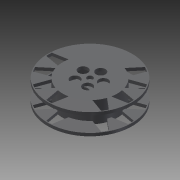
# Autodesk Inventor part: Wheel
Saved by Autodesk Inventor 2014 SP1 (Build 180222100, 222)
## iProperties
Created: 2014-11-21
Part Number: Wheel
Material: Generic
Document SubType Name: Modeling
Designer: AlecShufelt
Density: 1 g/cm^3
Appearance: Smooth - Medium Gray
Author: AlecShufelt
Autodesk Inventor part; units mm, degrees
ref_plane "YZ Plane" through (0, 0, 0) normal (1, 0, 0) x (0, 1, 0)
ref_plane "XZ Plane" through (0, 0, 0) normal (0, 1, 0) x (-1, 0, 0)
ref_plane "XY Plane" through (0, 0, 0) normal (0, 0, 1) x (1, 0, 0)
sketch "Sketch1" plane through (0, 0, 0) normal (0, 1, 0) x (-1, 0, 0)
  circle A0 centre (0, 0) radius 114.3
  dimension "d0" = 228.6
  constraints: 1 centre point, 1 coincident
  measures "d0" diameter of A0
extrude "Extrusion1" add sketch "Sketch1" along normal blind 7.9756
sketch "Sketch2" plane through (0, 7.9756, 0) normal (0, 1, 0) x (1, 0, 0)
  circle A0 centre (0, 0) radius 114.3 projected
  circle A1 centre (0, 0) radius 74.2569
  dimension "d3" = 148.5138
  constraints: 1 centre point, 1 coincident
  measures "d3" diameter of A1
extrude "Extrusion2" add sketch "Sketch2" along normal blind 41.0464 contours A1
sketch "Sketch3" plane through (0, 49.022, 0) normal (0, 1, 0) x (1, 0, 0)
  circle A0 centre (0, 0) radius 74.2569 projected
  circle A1 centre (0, 0) radius 114.3
  dimension "d6" = 228.6
  constraints: 1 centre point, 1 coincident
  measures "d6" diameter of A1
extrude "Extrusion3" add sketch "Sketch3" along normal blind 7.9756 contours A0 | A1
sketch "Sketch4" plane through (0, 56.9976, 0) normal (0, 1, 0) x (1, 0, 0)
  circle A0 centre (0, 0) radius 114.3 projected
  circle A1 centre (0, 0) radius 111.76
  circle A2 centre (0, 0) radius 74.2569
  line L0 (14.605, 72.8065) -> (7.62, 111.4999)
  line L1 (-14.605, 72.8065) -> (-7.62, 111.4999)
  line L2 (0, 0) -> (0, 82.3144)
  circle A3 centre (0, 0) radius 111.76
  circle A4 centre (0, 0) radius 74.2569
  line L3 (-23.7549, 70.3547) -> (-49.1508, 100.3718)
  line L4 (-49.0515, 55.7497) -> (-62.3491, 92.7518)
  circle A5 centre (0, 0) radius 111.76
  circle A6 centre (0, 0) radius 74.2569
  line L5 (-55.7497, 49.0515) -> (-92.7518, 62.3491)
  line L6 (-70.3547, 23.7549) -> (-100.3718, 49.1508)
  circle A7 centre (0, 0) radius 111.76
  circle A8 centre (0, 0) radius 74.2569
  line L7 (-72.8065, 14.605) -> (-111.4999, 7.62)
  line L8 (-72.8065, -14.605) -> (-111.4999, -7.62)
  circle A9 centre (0, 0) radius 111.76
  circle A10 centre (0, 0) radius 74.2569
  line L9 (-70.3547, -23.7549) -> (-100.3718, -49.1508)
  line L10 (-55.7497, -49.0515) -> (-92.7518, -62.3491)
  circle A11 centre (0, 0) radius 111.76
  circle A12 centre (0, 0) radius 74.2569
  line L11 (-49.0515, -55.7497) -> (-62.3491, -92.7518)
  line L12 (-23.7549, -70.3547) -> (-49.1508, -100.3718)
  circle A13 centre (0, 0) radius 111.76
  circle A14 centre (0, 0) radius 74.2569
  line L13 (-14.605, -72.8065) -> (-7.62, -111.4999)
  line L14 (14.605, -72.8065) -> (7.62, -111.4999)
  circle A15 centre (0, 0) radius 111.76
  circle A16 centre (0, 0) radius 74.2569
  line L15 (23.7549, -70.3547) -> (49.1508, -100.3718)
  line L16 (49.0515, -55.7497) -> (62.3491, -92.7518)
  circle A17 centre (0, 0) radius 111.76
  circle A18 centre (0, 0) radius 74.2569
  line L17 (55.7497, -49.0515) -> (92.7518, -62.3491)
  line L18 (70.3547, -23.7549) -> (100.3718, -49.1508)
  circle A19 centre (0, 0) radius 111.76
  circle A20 centre (0, 0) radius 74.2569
  line L19 (72.8065, -14.605) -> (111.4999, -7.62)
  line L20 (72.8065, 14.605) -> (111.4999, 7.62)
  circle A21 centre (0, 0) radius 111.76
  circle A22 centre (0, 0) radius 74.2569
  line L21 (70.3547, 23.7549) -> (100.3718, 49.1508)
  line L22 (55.7497, 49.0515) -> (92.7518, 62.3491)
  circle A23 centre (0, 0) radius 111.76
  circle A24 centre (0, 0) radius 74.2569
  line L23 (49.0515, 55.7497) -> (62.3491, 92.7518)
  line L24 (23.7549, 70.3547) -> (49.1508, 100.3718)
  dimension "d10" = 148.5138
  dimension "d11" = 29.21
  dimension "d12" = 14.605
  dimension "d13" = 15.24
  dimension "d14" = 7.62
  dimension "d17" = 360
  constraints: 50 end point, 48 point on circle, 26 coincident, 24 centre point, 1 vertical, 131 other
  measures "d10" diameter of A2
  measures "d11" distance of L0.start L1.start
  measures "d12" distance from line of L2 L1.start
  measures "d13" distance of L0.end L1.end
  measures "d14" distance from line of L2 L1.end
extrude "Extrusion4" cut sketch "Sketch4" against normal blind 12700 contours A1 L19 A2 L20 | L21 A2 L22 A1 | A1 L17 A2 L18 | L23 A2 L24 A1 | A1 L13 A2 L14 | A1 L11 A2 L12 | A1 L9 A2 L10 | L7 A2 L8 A1
sketch "Sketch5" plane through (0, 56.9976, 0) normal (0, 1, 0) x (1, 0, 0)
  arc A0 (100.3718, 49.1508) -> (92.7518, 62.3491) centre (0, 0) ccw projected
  circle A1 centre (0, 29.1163) radius 12.7
  circle A2 centre (-27.6912, 8.9974) radius 12.7
  circle A3 centre (-17.1141, -23.5556) radius 12.7
  circle A4 centre (17.1141, -23.5556) radius 12.7
  circle A5 centre (27.6912, 8.9974) radius 12.7
  dimension "d21" = 25.4
  dimension "d24" = 360
  constraints: 5 centre point, 11 other
  measures "d21" diameter of A1
extrude "Extrusion5" cut sketch "Sketch5" against normal blind 12700
sketch "Sketch6" plane through (0, 49.022, 0) normal (0, -1, 0) x (1, 0, 0)
  arc A0 (70.3547, -23.7549) -> (72.8065, -14.605) centre (0, 0) ccw projected
  circle A1 centre (0, 0) radius 70.5777
  constraints: 1 centre point, 1 coincident
extrude "Extrusion6" cut sketch "Sketch6" along normal blind 41.021
sketch "Sketch7" plane through (0, 0, 0) normal (0, -1, 0) x (1, 0, 0)
  circle A0 centre (0, 0) radius 114.3 projected
  circle A1 centre (0, 0) radius 7.62
  dimension "d30" = 15.24
  constraints: 1 centre point, 1 coincident
  measures "d30" diameter of A1
extrude "Extrusion7" cut sketch "Sketch7" against normal blind 174.879 contours A1
body "Solid1"
